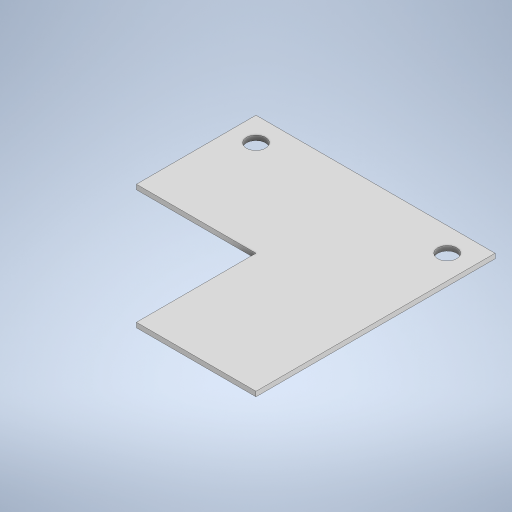
# Autodesk Inventor part: Pinz
Saved by Autodesk Inventor 2023 (Build 270158000, 158)
## iProperties
Created: 2022-11-06
Part Number: Pinz
Material: Generic
Document SubType Name: Modeling
Designer: SAMJ
Density: 1 g/cm^3
Appearance: Default
Author: SAMJ
Autodesk Inventor part; units mm, degrees
ref_plane "YZ Plane" through (0, 0, 0) normal (1, 0, 0) x (0, 1, 0)
ref_plane "XZ Plane" through (0, 0, 0) normal (0, 1, 0) x (-1, 0, 0)
ref_plane "XY Plane" through (0, 0, 0) normal (0, 0, 1) x (1, 0, 0)
sketch "Sketch1" plane through (0, 0, 0) normal (0, 1, 0) x (-1, 0, 0)
  line L0 (-50, 25) -> (50, 25)
  line L1 (50, 25) -> (50, -25)
  line L2 (50, -25) -> (-50, -25)
  line L3 (-50, -25) -> (-50, 25)
  line L4 (-50, 25) -> (0, 25)
  line L5 (0, 25) -> (0, 75)
  line L6 (0, 75) -> (-50, 75)
  line L7 (-50, 75) -> (-50, 25)
  line L8 (50, -25) -> (40, -25)
  line L9 (40, -25) -> (40, -15)
  line L10 (-50, -25) -> (-50, -15)
  line L11 (-50, -15) -> (-40, -15)
  circle A0 centre (40, -15) radius 4
  circle A1 centre (-40, -15) radius 4
  point P0 (0, 0)
  point P1 (0, 25)
  dimension "d0" = 100
  dimension "d1" = 50
  dimension "d2" = 50
  dimension "d3" = 50
  dimension "d4" = 10
  dimension "d5" = 10
  dimension "d6" = 10
  dimension "d7" = 10
  dimension "d8" = 8
  dimension "d9" = 8
  dimension "d12" = 90
  dimension "d13" = 90
  constraints: 24 end point, 4 parallel, 2 centre point, 2 coincident, 2 horizontal, 2 perpendicular, 2 point on line
  measures "d0" distance of L1.end L2.end
  measures "d1" distance of L0.end L1.end
  measures "d2" distance of L6.end L5.end
  measures "d3" distance of L5.end L4.end
  measures "d4" distance of L1.end L8.end
  measures "d5" distance of L8.end L9.end
  measures "d6" distance of L2.end L10.end
  measures "d7" distance of L10.end L11.end
  measures "d8" diameter of A0
  measures "d9" diameter of A1
  measures "d12" angle of L9 L2
  measures "d13" angle of L10 L11
extrude "Extrusion1" add sketch "Sketch1" along normal blind 2
body "Solid1"
